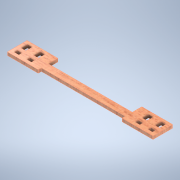
# Autodesk Inventor part: DoorFrameTop_V3
Saved by Autodesk Inventor 2022.2 (Build 262287000, 287)
## iProperties
Created: 2023-03-05
Part Number: DoorFrameTop_V3
Material: Wood (Oak)
Document SubType Name: Modeling
Designer: jaege
Density: 0.76 g/cm^3
Appearance: Red Oak - Natural Low Gloss
Author: jaege
Autodesk Inventor part; units mm, degrees
ref_plane "YZ Plane" through (0, 0, 0) normal (1, 0, 0) x (0, 1, 0)
ref_plane "XZ Plane" through (0, 0, 0) normal (0, 1, 0) x (-1, 0, 0)
ref_plane "XY Plane" through (0, 0, 0) normal (0, 0, 1) x (1, 0, 0)
sketch "Sketch1" plane through (0, 0, 0) normal (0, 1, 0) x (-1, 0, 0)
  line L0 (92, -24.95) -> (53, -24.95)
  line L1 (53, 0) -> (92, 0)
  line L2 (92, 0) -> (92, -24.95)
  line L3 (53, -24.95) -> (53, 0) construction
  line L4 (0, -24.95) -> (0, 0) construction
  line L5 (92, -8) -> (0, -8) construction
  line L6 (92, -4) -> (0, -4) construction
  line L7 (92, -20.95) -> (0, -20.95) construction
  line L8 (53, -24.95) -> (53, -12.9)
  line L9 (92, -12.9) -> (0, -12.9) construction
  line L10 (92, -24.95) -> (0, -24.95) construction
  line L11 (87.5, -24.95) -> (87.5, 0) construction
  line L12 (71.5, -24.95) -> (71.5, 0) construction
  line L13 (65.5, -24.95) -> (65.5, 0) construction
  line L14 (81.5, 0) -> (81.5, -24.95) construction
  line L15 (87.5, -20.95) -> (81.5, -20.95)
  line L16 (81.5, -20.95) -> (81.5, -12.9)
  line L17 (81.5, -12.9) -> (87.5, -12.9)
  line L18 (87.5, -12.9) -> (87.5, -20.95)
  line L19 (71.5, -20.95) -> (65.5, -20.95)
  line L20 (65.5, -20.95) -> (65.5, -12.9)
  line L21 (65.5, -12.9) -> (71.5, -12.9)
  line L22 (71.5, -12.9) -> (71.5, -20.95)
  line L23 (71.5, -8) -> (65.5, -8)
  line L24 (65.5, -8) -> (65.5, -4)
  line L25 (65.5, -4) -> (71.5, -4)
  line L26 (71.5, -4) -> (71.5, -8)
  line L27 (87.5, -8) -> (81.5, -8)
  line L28 (81.5, -8) -> (81.5, -4)
  line L29 (81.5, -4) -> (87.5, -4)
  line L30 (87.5, -4) -> (87.5, -8)
  line L31 (53, -12.9) -> (0, -12.9)
  line L32 (92, 0) -> (0, 0) construction
  line L33 (53, 0) -> (53, -4)
  line L34 (53, -4) -> (0, -4)
  line L35 (-92, -24.95) -> (-53, -24.95)
  line L36 (-53, 0) -> (-92, 0)
  line L37 (-92, 0) -> (-92, -24.95)
  line L38 (-53, -24.95) -> (-53, 0) construction
  line L39 (-92, -8) -> (0, -8) construction
  line L40 (-92, -4) -> (0, -4) construction
  line L41 (-92, -20.95) -> (0, -20.95) construction
  line L42 (-53, -24.95) -> (-53, -12.9)
  line L43 (-92, -12.9) -> (0, -12.9) construction
  line L44 (-92, -24.95) -> (0, -24.95) construction
  line L45 (-87.5, -24.95) -> (-87.5, 0) construction
  line L46 (-71.5, -24.95) -> (-71.5, 0) construction
  line L47 (-65.5, -24.95) -> (-65.5, 0) construction
  line L48 (-81.5, 0) -> (-81.5, -24.95) construction
  line L49 (-87.5, -20.95) -> (-81.5, -20.95)
  line L50 (-81.5, -20.95) -> (-81.5, -12.9)
  line L51 (-81.5, -12.9) -> (-87.5, -12.9)
  line L52 (-87.5, -12.9) -> (-87.5, -20.95)
  line L53 (-71.5, -20.95) -> (-65.5, -20.95)
  line L54 (-65.5, -20.95) -> (-65.5, -12.9)
  line L55 (-65.5, -12.9) -> (-71.5, -12.9)
  line L56 (-71.5, -12.9) -> (-71.5, -20.95)
  line L57 (-71.5, -8) -> (-65.5, -8)
  line L58 (-65.5, -8) -> (-65.5, -4)
  line L59 (-65.5, -4) -> (-71.5, -4)
  line L60 (-71.5, -4) -> (-71.5, -8)
  line L61 (-87.5, -8) -> (-81.5, -8)
  line L62 (-81.5, -8) -> (-81.5, -4)
  line L63 (-81.5, -4) -> (-87.5, -4)
  line L64 (-87.5, -4) -> (-87.5, -8)
  line L65 (-53, -12.9) -> (0, -12.9)
  line L66 (-92, 0) -> (0, 0) construction
  line L67 (-53, 0) -> (-53, -4)
  line L68 (-53, -4) -> (0, -4)
  dimension "d19" = 8.05
  dimension "d20" = 4
  dimension "d21" = 4.9
  dimension "d22" = 4
  dimension "d24" = 6
  dimension "d25" = 10
  dimension "d26" = 6
  dimension "d27" = 12.5
  dimension "d28" = 4.5
  dimension "d29" = 92
  dimension "d30" = 4
  constraints: 139 end point, 67 point on line, 34 symmetric about line, 9 parallel, 9 perpendicular, 7 horizontal, 2 collinear, 2 vertical
  measures "d19" distance between parallel lines of L9 L7
  measures "d20" distance between parallel lines of L10 L7
  measures "d21" distance between parallel lines of L5 L9
  measures "d22" distance between parallel lines of L6 L5
  measures "d24" distance between parallel lines of L14 L11
  measures "d25" distance between parallel lines of L12 L14
  measures "d26" distance between parallel lines of L13 L12
  measures "d27" distance between parallel lines of L8 L13
  measures "d28" distance between parallel lines of L2 L11
  measures "d29" distance of L4.start L0.start
  measures "d30" distance between parallel lines of L32 L6
extrude "Extrusion1" add sketch "Sketch1" along normal blind 4
body "Solid1"
